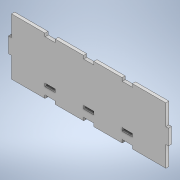
# Autodesk Inventor part: Стенка t1
Saved by Autodesk Inventor 2021 (Build 250183000, 183)
## iProperties
Created: 2021-04-11
Part Number: Стенка t1
Material: Типовые
Document SubType Name: Modeling
Designer: user
Density: 1 g/cm^3
Appearance: По умолчанию
Author: user
Autodesk Inventor part; units mm, degrees
ref_plane "YZ Plane" through (0, 0, 0) normal (1, 0, 0) x (0, 1, 0)
ref_plane "XZ Plane" through (0, 0, 0) normal (0, 1, 0) x (-1, 0, 0)
ref_plane "XY Plane" through (0, 0, 0) normal (0, 0, 1) x (1, 0, 0)
sketch "Эскиз1" plane through (0, 0, 0) normal (0, 0, 1) x (1, 0, 0)
  line L0 (-32.5, -22.5) -> (-32.5, -19.5)
  line L1 (-32.5, -19.5) -> (-42.5, -19.5)
  line L2 (-42.5, -19.5) -> (-42.5, -22.5)
  line L3 (0, -19.5) -> (-5, -19.5)
  line L4 (-5, -19.5) -> (-5, -22.5)
  line L5 (-75, 22.5) -> (-42.5, 22.5)
  line L6 (-32.5, 22.5) -> (-32.5, 19.5)
  line L7 (-32.5, 19.5) -> (-42.5, 19.5)
  line L8 (-42.5, 19.5) -> (-42.5, 22.5)
  line L9 (-32.5, 22.5) -> (-5, 22.5)
  line L10 (0, 19.5) -> (-5, 19.5)
  line L11 (-5, 19.5) -> (-5, 22.5)
  line L12 (-5, 22.5) -> (-32.5, 22.5)
  line L13 (-42.5, 22.5) -> (-75, 22.5)
  line L14 (32.5, -22.5) -> (32.5, -19.5)
  line L15 (32.5, -19.5) -> (42.5, -19.5)
  line L16 (42.5, -19.5) -> (42.5, -22.5)
  line L17 (0, -19.5) -> (5, -19.5)
  line L18 (5, -19.5) -> (5, -22.5)
  line L19 (75, 22.5) -> (42.5, 22.5)
  line L20 (32.5, 22.5) -> (32.5, 19.5)
  line L21 (32.5, 19.5) -> (42.5, 19.5)
  line L22 (42.5, 19.5) -> (42.5, 22.5)
  line L23 (32.5, 22.5) -> (5, 22.5)
  line L24 (0, 19.5) -> (5, 19.5)
  line L25 (5, 19.5) -> (5, 22.5)
  line L26 (5, 22.5) -> (32.5, 22.5)
  line L27 (42.5, 22.5) -> (75, 22.5)
  line L28 (-42.5, -22.5) -> (-32.5, -22.5)
  line L29 (-5, -22.5) -> (5, -22.5)
  line L30 (32.5, -22.5) -> (42.5, -22.5)
  line L31 (-32.5, -32.5) -> (-32.5, -29.5)
  line L32 (-32.5, -29.5) -> (-42.5, -29.5)
  line L33 (-42.5, -29.5) -> (-42.5, -32.5)
  line L34 (5, -32.5) -> (5, -29.5)
  line L35 (5, -29.5) -> (-5, -29.5)
  line L36 (-5, -29.5) -> (-5, -32.5)
  line L37 (42.5, -32.5) -> (42.5, -29.5)
  line L38 (42.5, -29.5) -> (32.5, -29.5)
  line L39 (32.5, -29.5) -> (32.5, -32.5)
  line L40 (-75, 2.5) -> (-78, 2.5)
  line L41 (-78, 2.5) -> (-78, -12.5)
  line L42 (-78, -12.5) -> (-75, -12.5)
  line L43 (77.5, 2.5) -> (75, 2.5)
  line L44 (75, -12.5) -> (77.5, -12.5)
  line L45 (77.5, -12.5) -> (77.5, 2.5)
  line L46 (75, -32.5) -> (42.5, -32.5)
  line L47 (32.5, -32.5) -> (5, -32.5)
  line L48 (-5, -32.5) -> (-32.5, -32.5)
  line L49 (-42.5, -32.5) -> (-75, -32.5)
  line L50 (-75, 22.5) -> (-75, 2.5)
  line L51 (-75, -12.5) -> (-75, -32.5)
  line L52 (75, 22.5) -> (75, 2.5)
  line L53 (75, -12.5) -> (75, -32.5)
  point P0 (0, 0)
  constraints: 108 end point, 12 equal length, 9 perpendicular, 3 horizontal, 1 point on line
extrude "Выдавливание2" add sketch "Эскиз1" along normal blind 3
